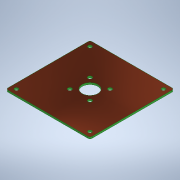
# Autodesk Inventor part: pcb
Saved by Autodesk Inventor 2022 (Build 260153000, 153)
## iProperties
Created: 2022-04-25
Part Number: pcb
Material: Generic
Document SubType Name: Modeling
Designer: Bowen
Density: 1 g/cm^3
Appearance: Smooth - Dark Forest Green
Author: Bowen
Autodesk Inventor part; units mm, degrees
ref_plane "YZ Plane" through (0, 0, 0) normal (1, 0, 0) x (0, 1, 0)
ref_plane "XZ Plane" through (0, 0, 0) normal (0, 1, 0) x (-1, 0, 0)
ref_plane "XY Plane" through (0, 0, 0) normal (0, 0, 1) x (1, 0, 0)
sketch "Sketch1" plane through (0, 0, 0) normal (0, 1, 0) x (-1, 0, 0)
  line L0 (40, -40) -> (-40, -40)
  line L1 (-40, -40) -> (-40, 40)
  line L2 (-40, 40) -> (40, 40)
  line L3 (40, 40) -> (40, -40)
  point P0 (0, 0)
  point P1 (0, -40)
  point P2 (-40, 0)
  dimension "d15" = 80
  dimension "d16" = 80
  constraints: 8 end point, 2 midpoint, 2 parallel, 1 horizontal, 1 horizontal alignment, 1 perpendicular, 1 vertical alignment
  measures "d15" distance of L0.start L0.end
  measures "d16" distance of L0.end L1.end
extrude "Extrusion1" add sketch "Sketch1" along normal mid plane 1.6
fillet "Fillet1" radius 2 4 edges at (-40, 0, 40) (40, 0, 40) (40, 0, -40) (-40, 0, -40)
sketch "Sketch2" plane through (0, 0.8, 0) normal (0, 1, 0) x (1, 0, 0)
  line L0 (0, 0) -> (-7.9877, 0) construction
  line L1 (0, 0) -> (0, 5.5351) construction
  point P0 (-35, -35)
  point P1 (-35, 35)
  point P2 (35, -35)
  point P3 (35, 35)
  dimension "d18" = 35
  dimension "d19" = 35
  constraints: 4 end point, 3 symmetric about line, 1 horizontal, 1 vertical
  measures "d18" horizontal distance of L0.start point (-35, -35)
  measures "d19" horizontal distance of L0.start point (-35, -35)
hole "Hole1" at (-35, 0.8, 35) at (-35, 0.8, -35) at (35, 0.8, 35) at (35, 0.8, -35) direction (0, -1, 0) diameter 3.454 end through all clearance for "Flat Head Machine Screw (82)" size "#4" standard "Ansi Unified Screw Threads"
sketch "Sketch3" plane through (0, 0.8, 0) normal (0, 1, 0) x (1, 0, 0)
  line L0 (-12.55, 12.55) -> (12.55, 12.55)
  line L1 (12.55, 12.55) -> (12.55, -12.55)
  line L2 (12.55, -12.55) -> (-12.55, -12.55)
  line L3 (-12.55, -12.55) -> (-12.55, 12.55)
  line L4 (0, 0) -> (0, 3.6765) construction
  line L5 (0, 0) -> (3.2883, 0) construction
  point P0 (12.55, 0)
  point P1 (0, 12.55)
  point P2 (-9.55, 9.55)
  point P3 (9.55, 9.55)
  point P4 (-9.55, -9.55)
  point P5 (9.55, -9.55)
  dimension "d27" = 25.1
  dimension "d28" = 25.1
  dimension "d29" = 3
  dimension "d30" = 3
  constraints: 12 end point, 3 symmetric about line, 2 horizontal, 2 midpoint, 2 parallel, 1 horizontal alignment, 1 perpendicular, 1 vertical, 1 vertical alignment
  measures "d27" distance of L1.end L2.end
  measures "d28" distance of L0.end L1.end
  measures "d29" distance from line of L0 point (-9.55, 9.55)
  measures "d30" distance from line of L3 point (-9.55, 9.55)
hole "Hole2" at (-9.55, 0.8, -9.55) at (9.55, 0.8, -9.55) at (-9.55, 0.8, 9.55) at (9.55, 0.8, 9.55) direction (0, -1, 0) diameter 3.7 end through all
sketch "Sketch4" plane through (0, 0.8, 0) normal (0, 1, 0) x (1, 0, 0)
  circle A0 centre (0, 0) radius 7.5
  dimension "d38" = 15
  constraints: 1 centre point, 1 coincident
  measures "d38" diameter of A0
extrude "Extrusion2" cut sketch "Sketch4" against normal through all
body "Solid1"
